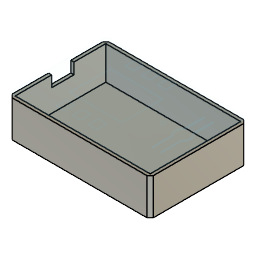
hamba gaming consol back shell (Autodesk Fusion 360 design; units mm, degrees)
Autodesk Fusion 360 part; units mm, degrees
sketch "Sketch1" plane through (0, 0, 0) normal (0, 0, 1) x (1, 0, 0)
  line L0 (0, 0) -> (83, 0)
  line L1 (83, 0) -> (83, 55)
  line L2 (83, 55) -> (0, 55)
  line L3 (0, 55) -> (0, 0)
  dimension "d1" = 83
  dimension "d2" = 55
  constraint horizontal L0
  constraint vertical L1
  constraint horizontal L2
  constraint vertical L3
  constraint coincident L0.start L3.end
  measures "d1" distance of L0.start L0.end
  measures "d2" distance of L0.start L2.end
extrude "Extrude1" add sketch "Sketch1" along normal blind 10 makes body 1
sketch "Sketch2" plane through (0, 0, 10) normal (0, 0, 1) x (-1, 0, 0)
  line L0 (0, -55) -> (0, 0)
  line L1 (0, 0) -> (-83, 0)
  line L2 (-83, 0) -> (-83, -55)
  line L3 (-83, -55) -> (0, -55)
  line L4 (-49, -42) -> (-49, -37.6986)
  line L5 (-49, -37.6986) -> (-52.5265, -34.3884)
  line L6 (-52.5265, -34.3884) -> (-52.5265, -24)
  line L7 (-52.5265, -24) -> (-49, -20.2432)
  line L8 (-49, -20.2432) -> (-49, -16)
  line L9 (-49, -16) -> (-2, -16)
  line L10 (-2, -16) -> (-0.5319, -18.1216)
  line L11 (-0.5319, -18.1216) -> (-0.5319, -23)
  line L12 (-0.5319, -23) -> (-1.2659, -24.8699)
  line L13 (-1.2659, -24.8699) -> (-1.2659, -33)
  line L14 (-1.2659, -33) -> (-0.5319, -34.4212)
  line L15 (-0.5319, -34.4212) -> (-0.5319, -39.5049)
  line L16 (-0.5319, -39.5049) -> (-3.3048, -42.6926)
  line L17 (-3.3048, -42.6926) -> (-49, -42)
  constraint perpendicular L5 L7
  constraint parallel L6 L8
  constraint perpendicular L0 L9
  constraint perpendicular L9 L11
  constraint parallel L11 L13
  constraint parallel L13 L15
  constraint vertical L4
extrude "Extrude2" add sketch "Sketch2" along normal blind 6 contours L4 L5 L6 L7 L8 L9 L10 L11 L12 L13 L14 L15 L16 L17 bodies 1
sketch "Sketch3" plane through (0, 0, 16) normal (0, 0, 1) x (-1, 0, 0)
  line L0 (-3.3048, -42.6926) -> (-0.5319, -39.5049)
  line L1 (-0.5319, -39.5049) -> (-0.5319, -34.4212)
  line L2 (-0.5319, -34.4212) -> (-1.2659, -33)
  line L3 (-1.2659, -33) -> (-1.2659, -24.8699)
  line L4 (-1.2659, -24.8699) -> (-0.5319, -23)
  line L5 (-0.5319, -23) -> (-0.5319, -18.1216)
  line L6 (-0.5319, -18.1216) -> (-2, -16)
  line L7 (-2, -16) -> (-49, -16)
  line L8 (-49, -16) -> (-49, -20.2432)
  line L9 (-49, -20.2432) -> (-52.5265, -24)
  line L10 (-52.5265, -24) -> (-52.5265, -34.3884)
  line L11 (-52.5265, -34.3884) -> (-49, -37.6986)
  line L12 (-49, -37.6986) -> (-49, -42)
  line L13 (-49, -42) -> (-3.3048, -42.6926)
  line L14 (-46, -38) -> (-20, -38)
  line L15 (-20, -38) -> (-20, -20)
  line L16 (-20, -20) -> (-46, -20)
  line L17 (-46, -20) -> (-46, -38)
  constraint horizontal L14
  constraint vertical L15
  constraint horizontal L16
  constraint vertical L17
extrude "Extrude3" add sketch "Sketch3" along normal blind 5 contours L14 L15 L16 L17 bodies 1
sketch "Sketch4" plane through (0, 0, 16) normal (0, 0, 1) x (-1, 0, 0)
  line L0 (-46, -20) -> (-20, -20)
  line L1 (-20, -20) -> (-20, -38)
  line L2 (-20, -38) -> (-46, -38)
  line L3 (-46, -38) -> (-46, -20)
  line L4 (-3.3048, -42.6926) -> (-0.5319, -39.5049)
  line L5 (-0.5319, -39.5049) -> (-0.5319, -34.4212)
  line L6 (-0.5319, -34.4212) -> (-1.2659, -33)
  line L7 (-1.2659, -33) -> (-1.2659, -24.8699)
  line L8 (-1.2659, -24.8699) -> (-0.5319, -23)
  line L9 (-0.5319, -23) -> (-0.5319, -18.1216)
  line L10 (-0.5319, -18.1216) -> (-2, -16)
  line L11 (-2, -16) -> (-49, -16)
  line L12 (-49, -16) -> (-49, -20.2432)
  line L13 (-49, -20.2432) -> (-52.5265, -24)
  line L14 (-52.5265, -24) -> (-52.5265, -34.3884)
  line L15 (-52.5265, -34.3884) -> (-49, -37.6986)
  line L16 (-49, -37.6986) -> (-49, -42)
  line L17 (-49, -42) -> (-3.3048, -42.6926)
  line L18 (-1.2659, -33) -> (-7, -33)
  line L19 (-7, -33) -> (-7, -25)
  line L20 (-7, -25) -> (-1.2659, -25)
  line L21 (-1.2659, -25) -> (-1.2659, -33)
  constraint horizontal L18
  constraint vertical L19
  constraint horizontal L20
  constraint vertical L21
  constraint coincident L6.end L7.start
extrude "Extrude4" add sketch "Sketch4" along normal blind 2 contours L7 L18 L19 L20 L21 bodies 1
sketch "Sketch5" plane through (0, 0, 10) normal (0, 0, 1) x (-1, 0, 0)
  line L0 (-3.3048, -42.6926) -> (-49, -42)
  line L1 (-49, -42) -> (-49, -37.6986)
  line L2 (-49, -37.6986) -> (-52.5265, -34.3884)
  line L3 (-52.5265, -34.3884) -> (-52.5265, -24)
  line L4 (-52.5265, -24) -> (-49, -20.2432)
  line L5 (-49, -20.2432) -> (-49, -16)
  line L6 (-49, -16) -> (-2, -16)
  line L7 (-2, -16) -> (-0.5319, -18.1216)
  line L8 (-0.5319, -18.1216) -> (-0.5319, -23)
  line L9 (-0.5319, -23) -> (-1.2659, -24.8699)
  line L10 (-1.2659, -24.8699) -> (-1.2659, -33)
  line L11 (-1.2659, -33) -> (-0.5319, -34.4212)
  line L12 (-0.5319, -34.4212) -> (-0.5319, -39.5049)
  line L13 (-0.5319, -39.5049) -> (-3.3048, -42.6926)
  line L14 (0, -55) -> (0, 0)
  line L15 (0, 0) -> (-83, 0)
  line L16 (-83, 0) -> (-83, -55)
  line L17 (-83, -55) -> (0, -55)
  line L18 (-43.127, -5.4877) -> (-41.627, -5.4877)
  line L19 (-40.877, -6.2377) -> (-40.877, -8.8377)
  line L20 (-41.627, -9.5877) -> (-43.127, -9.5877)
  line L21 (-43.877, -8.8377) -> (-43.877, -6.2377)
  arc A0 (-43.127, -5.4877) -> (-43.877, -6.2377) centre (-43.127, -6.2377) ccw
  arc A1 (-40.877, -6.2377) -> (-41.627, -5.4877) centre (-41.627, -6.2377) ccw
  arc A2 (-41.627, -9.5877) -> (-40.877, -8.8377) centre (-41.627, -8.8377) ccw
  arc A3 (-43.877, -8.8377) -> (-43.127, -9.5877) centre (-43.127, -8.8377) ccw
  arc A4 (-31.377, -9.5877) -> (-30.627, -8.8377) centre (-31.377, -8.8377) ccw
  line L22 (-31.377, -9.5877) -> (-32.877, -9.5877)
  arc A5 (-33.627, -8.8377) -> (-32.877, -9.5877) centre (-32.877, -8.8377) ccw
  line L23 (-33.627, -8.8377) -> (-33.627, -6.2377)
  arc A6 (-32.877, -5.4877) -> (-33.627, -6.2377) centre (-32.877, -6.2377) ccw
  line L24 (-32.877, -5.4877) -> (-31.377, -5.4877)
  arc A7 (-30.627, -6.2377) -> (-31.377, -5.4877) centre (-31.377, -6.2377) ccw
  line L25 (-30.627, -6.2377) -> (-30.627, -8.8377)
  arc A8 (-21.127, -9.5877) -> (-20.377, -8.8377) centre (-21.127, -8.8377) ccw
  line L26 (-21.127, -9.5877) -> (-22.627, -9.5877)
  arc A9 (-23.377, -8.8377) -> (-22.627, -9.5877) centre (-22.627, -8.8377) ccw
  line L27 (-23.377, -8.8377) -> (-23.377, -6.2377)
  arc A10 (-22.627, -5.4877) -> (-23.377, -6.2377) centre (-22.627, -6.2377) ccw
  line L28 (-22.627, -5.4877) -> (-21.127, -5.4877)
  arc A11 (-20.377, -6.2377) -> (-21.127, -5.4877) centre (-21.127, -6.2377) ccw
  line L29 (-20.377, -6.2377) -> (-20.377, -8.8377)
  arc A12 (-41.627, -53.0877) -> (-40.877, -52.3377) centre (-41.627, -52.3377) ccw
  line L30 (-41.627, -53.0877) -> (-43.127, -53.0877)
  arc A13 (-43.877, -52.3377) -> (-43.127, -53.0877) centre (-43.127, -52.3377) ccw
  line L31 (-43.877, -52.3377) -> (-43.877, -49.7377)
  arc A14 (-43.127, -48.9877) -> (-43.877, -49.7377) centre (-43.127, -49.7377) ccw
  line L32 (-43.127, -48.9877) -> (-41.627, -48.9877)
  arc A15 (-40.877, -49.7377) -> (-41.627, -48.9877) centre (-41.627, -49.7377) ccw
  line L33 (-40.877, -49.7377) -> (-40.877, -52.3377)
  arc A16 (-31.377, -53.0877) -> (-30.627, -52.3377) centre (-31.377, -52.3377) ccw
  line L34 (-31.377, -53.0877) -> (-32.877, -53.0877)
  arc A17 (-33.627, -52.3377) -> (-32.877, -53.0877) centre (-32.877, -52.3377) ccw
  line L35 (-33.627, -52.3377) -> (-33.627, -49.7377)
  arc A18 (-32.877, -48.9877) -> (-33.627, -49.7377) centre (-32.877, -49.7377) ccw
  line L36 (-32.877, -48.9877) -> (-31.377, -48.9877)
  arc A19 (-30.627, -49.7377) -> (-31.377, -48.9877) centre (-31.377, -49.7377) ccw
  line L37 (-30.627, -49.7377) -> (-30.627, -52.3377)
  arc A20 (-21.127, -53.0877) -> (-20.377, -52.3377) centre (-21.127, -52.3377) ccw
  line L38 (-21.127, -53.0877) -> (-22.627, -53.0877)
  arc A21 (-23.377, -52.3377) -> (-22.627, -53.0877) centre (-22.627, -52.3377) ccw
  line L39 (-23.377, -52.3377) -> (-23.377, -49.7377)
  arc A22 (-22.627, -48.9877) -> (-23.377, -49.7377) centre (-22.627, -49.7377) ccw
  line L40 (-22.627, -48.9877) -> (-21.127, -48.9877)
  arc A23 (-20.377, -49.7377) -> (-21.127, -48.9877) centre (-21.127, -49.7377) ccw
  line L41 (-20.377, -49.7377) -> (-20.377, -52.3377)
  point P0 (-43.877, -5.4877)
  point P1 (-40.877, -5.4877)
  point P2 (-43.877, -9.5877)
  dimension "d11" = 3
  dimension "d12" = 4.1
  dimension "d13" = 0.75
  dimension "d16" = 20.5
  dimension "d17" = -43.5
  constraint horizontal L18
  constraint vertical L19
  constraint horizontal L20
  constraint vertical L21
  constraint coincident P0 L21
  constraint coincident P0 L18
  constraint tangent L21 A0
  constraint tangent L18 A0
  constraint coincident P1 L19
  constraint coincident P1 L18
  constraint tangent L19 A1
  constraint tangent L18 A1
  constraint equal A0 A1
  constraint tangent L20 A2
  constraint tangent L19 A2
  constraint equal A0 A2
  constraint coincident P2 L21
  constraint coincident P2 L20
  constraint tangent L21 A3
  constraint tangent L20 A3
  constraint equal A0 A3
  measures "d11" distance of P0 P1
  measures "d12" distance of P0 P2
  measures "d13" radius of A0
extrude "Extrude5" add sketch "Sketch5" along normal blind 10 contours L18 L19 L20 L21 A0 A1 A2 A3 | A4 L22 A5 L23 A6 L24 A7 L25 | A8 L26 A9 L27 A10 L28 A11 L29 | A12 L30 A13 L31 A14 L32 A15 L33 | A16 L34 A17 L35 A18 L36 A19 L37 | A20 L38 A21 L39 A22 L40 A23 L41 bodies 1
sketch "Sketch6" plane through (0, 0, 10) normal (0, 0, 1) x (-1, 0, 0)
  line L0 (-43.127, -48.9877) -> (-41.627, -48.9877)
  arc A0 (-40.877, -49.7377) -> (-41.627, -48.9877) centre (-41.627, -49.7377) ccw
  line L1 (-40.877, -49.7377) -> (-40.877, -52.3377)
  arc A1 (-41.627, -53.0877) -> (-40.877, -52.3377) centre (-41.627, -52.3377) ccw
  line L2 (-41.627, -53.0877) -> (-43.127, -53.0877)
  arc A2 (-43.877, -52.3377) -> (-43.127, -53.0877) centre (-43.127, -52.3377) ccw
  line L3 (-43.877, -52.3377) -> (-43.877, -49.7377)
  arc A3 (-43.127, -48.9877) -> (-43.877, -49.7377) centre (-43.127, -49.7377) ccw
  line L4 (-32.877, -5.4877) -> (-31.377, -5.4877)
  arc A4 (-30.627, -6.2377) -> (-31.377, -5.4877) centre (-31.377, -6.2377) ccw
  line L5 (-30.627, -6.2377) -> (-30.627, -8.8377)
  arc A5 (-31.377, -9.5877) -> (-30.627, -8.8377) centre (-31.377, -8.8377) ccw
  line L6 (-31.377, -9.5877) -> (-32.877, -9.5877)
  arc A6 (-33.627, -8.8377) -> (-32.877, -9.5877) centre (-32.877, -8.8377) ccw
  line L7 (-33.627, -8.8377) -> (-33.627, -6.2377)
  arc A7 (-32.877, -5.4877) -> (-33.627, -6.2377) centre (-32.877, -6.2377) ccw
  line L8 (-22.627, -5.4877) -> (-21.127, -5.4877)
  arc A8 (-20.377, -6.2377) -> (-21.127, -5.4877) centre (-21.127, -6.2377) ccw
  line L9 (-20.377, -6.2377) -> (-20.377, -8.8377)
  arc A9 (-21.127, -9.5877) -> (-20.377, -8.8377) centre (-21.127, -8.8377) ccw
  line L10 (-21.127, -9.5877) -> (-22.627, -9.5877)
  arc A10 (-23.377, -8.8377) -> (-22.627, -9.5877) centre (-22.627, -8.8377) ccw
  line L11 (-23.377, -8.8377) -> (-23.377, -6.2377)
  arc A11 (-22.627, -5.4877) -> (-23.377, -6.2377) centre (-22.627, -6.2377) ccw
  line L12 (-32.877, -48.9877) -> (-31.377, -48.9877)
  arc A12 (-30.627, -49.7377) -> (-31.377, -48.9877) centre (-31.377, -49.7377) ccw
  line L13 (-30.627, -49.7377) -> (-30.627, -52.3377)
  arc A13 (-31.377, -53.0877) -> (-30.627, -52.3377) centre (-31.377, -52.3377) ccw
  line L14 (-31.377, -53.0877) -> (-32.877, -53.0877)
  arc A14 (-33.627, -52.3377) -> (-32.877, -53.0877) centre (-32.877, -52.3377) ccw
  line L15 (-33.627, -52.3377) -> (-33.627, -49.7377)
  arc A15 (-32.877, -48.9877) -> (-33.627, -49.7377) centre (-32.877, -49.7377) ccw
  line L16 (-43.127, -5.4877) -> (-41.627, -5.4877)
  arc A16 (-40.877, -6.2377) -> (-41.627, -5.4877) centre (-41.627, -6.2377) ccw
  line L17 (-40.877, -6.2377) -> (-40.877, -8.8377)
  arc A17 (-41.627, -9.5877) -> (-40.877, -8.8377) centre (-41.627, -8.8377) ccw
  line L18 (-41.627, -9.5877) -> (-43.127, -9.5877)
  arc A18 (-43.877, -8.8377) -> (-43.127, -9.5877) centre (-43.127, -8.8377) ccw
  line L19 (-43.877, -8.8377) -> (-43.877, -6.2377)
  arc A19 (-43.127, -5.4877) -> (-43.877, -6.2377) centre (-43.127, -6.2377) ccw
  line L20 (-22.627, -48.9877) -> (-21.127, -48.9877)
  arc A20 (-20.377, -49.7377) -> (-21.127, -48.9877) centre (-21.127, -49.7377) ccw
  line L21 (-20.377, -49.7377) -> (-20.377, -52.3377)
  arc A21 (-21.127, -53.0877) -> (-20.377, -52.3377) centre (-21.127, -52.3377) ccw
  line L22 (-21.127, -53.0877) -> (-22.627, -53.0877)
  arc A22 (-23.377, -52.3377) -> (-22.627, -53.0877) centre (-22.627, -52.3377) ccw
  line L23 (-23.377, -52.3377) -> (-23.377, -49.7377)
  arc A23 (-22.627, -48.9877) -> (-23.377, -49.7377) centre (-22.627, -49.7377) ccw
  line L24 (-3.3048, -42.6926) -> (-49, -42)
  line L25 (-49, -42) -> (-49, -37.6986)
  line L26 (-49, -37.6986) -> (-52.5265, -34.3884)
  line L27 (-52.5265, -34.3884) -> (-52.5265, -24)
  line L28 (-52.5265, -24) -> (-49, -20.2432)
  line L29 (-49, -20.2432) -> (-49, -16)
  line L30 (-49, -16) -> (-2, -16)
  line L31 (-2, -16) -> (-0.5319, -18.1216)
  line L32 (-0.5319, -18.1216) -> (-0.5319, -23)
  line L33 (-0.5319, -23) -> (-1.2659, -24.8699)
  line L34 (-1.2659, -24.8699) -> (-1.2659, -33)
  line L35 (-1.2659, -33) -> (-0.5319, -34.4212)
  line L36 (-0.5319, -34.4212) -> (-0.5319, -39.5049)
  line L37 (-0.5319, -39.5049) -> (-3.3048, -42.6926)
  line L38 (0, -55) -> (0, 0)
  line L39 (0, 0) -> (-83, 0)
  line L40 (-83, 0) -> (-83, -55)
  line L41 (-83, -55) -> (0, -55)
  circle A24 centre (-62, -29) radius 6
  dimension "d20" = 12
  measures "d20" diameter of A24
extrude "Extrude6" add sketch "Sketch6" along normal blind 10 contours A24 bodies 1
sketch "Sketch7" plane through (0, 0, 10) normal (0, 0, 1) x (-1, 0, 0)
  circle A0 centre (-62, -29) radius 6
  line L0 (-43.127, -48.9877) -> (-41.627, -48.9877)
  arc A1 (-40.877, -49.7377) -> (-41.627, -48.9877) centre (-41.627, -49.7377) ccw
  line L1 (-40.877, -49.7377) -> (-40.877, -52.3377)
  arc A2 (-41.627, -53.0877) -> (-40.877, -52.3377) centre (-41.627, -52.3377) ccw
  line L2 (-41.627, -53.0877) -> (-43.127, -53.0877)
  arc A3 (-43.877, -52.3377) -> (-43.127, -53.0877) centre (-43.127, -52.3377) ccw
  line L3 (-43.877, -52.3377) -> (-43.877, -49.7377)
  arc A4 (-43.127, -48.9877) -> (-43.877, -49.7377) centre (-43.127, -49.7377) ccw
  line L4 (-32.877, -5.4877) -> (-31.377, -5.4877)
  arc A5 (-30.627, -6.2377) -> (-31.377, -5.4877) centre (-31.377, -6.2377) ccw
  line L5 (-30.627, -6.2377) -> (-30.627, -8.8377)
  arc A6 (-31.377, -9.5877) -> (-30.627, -8.8377) centre (-31.377, -8.8377) ccw
  line L6 (-31.377, -9.5877) -> (-32.877, -9.5877)
  arc A7 (-33.627, -8.8377) -> (-32.877, -9.5877) centre (-32.877, -8.8377) ccw
  line L7 (-33.627, -8.8377) -> (-33.627, -6.2377)
  arc A8 (-32.877, -5.4877) -> (-33.627, -6.2377) centre (-32.877, -6.2377) ccw
  line L8 (-22.627, -5.4877) -> (-21.127, -5.4877)
  arc A9 (-20.377, -6.2377) -> (-21.127, -5.4877) centre (-21.127, -6.2377) ccw
  line L9 (-20.377, -6.2377) -> (-20.377, -8.8377)
  arc A10 (-21.127, -9.5877) -> (-20.377, -8.8377) centre (-21.127, -8.8377) ccw
  line L10 (-21.127, -9.5877) -> (-22.627, -9.5877)
  arc A11 (-23.377, -8.8377) -> (-22.627, -9.5877) centre (-22.627, -8.8377) ccw
  line L11 (-23.377, -8.8377) -> (-23.377, -6.2377)
  arc A12 (-22.627, -5.4877) -> (-23.377, -6.2377) centre (-22.627, -6.2377) ccw
  line L12 (-32.877, -48.9877) -> (-31.377, -48.9877)
  arc A13 (-30.627, -49.7377) -> (-31.377, -48.9877) centre (-31.377, -49.7377) ccw
  line L13 (-30.627, -49.7377) -> (-30.627, -52.3377)
  arc A14 (-31.377, -53.0877) -> (-30.627, -52.3377) centre (-31.377, -52.3377) ccw
  line L14 (-31.377, -53.0877) -> (-32.877, -53.0877)
  arc A15 (-33.627, -52.3377) -> (-32.877, -53.0877) centre (-32.877, -52.3377) ccw
  line L15 (-33.627, -52.3377) -> (-33.627, -49.7377)
  arc A16 (-32.877, -48.9877) -> (-33.627, -49.7377) centre (-32.877, -49.7377) ccw
  line L16 (-43.127, -5.4877) -> (-41.627, -5.4877)
  arc A17 (-40.877, -6.2377) -> (-41.627, -5.4877) centre (-41.627, -6.2377) ccw
  line L17 (-40.877, -6.2377) -> (-40.877, -8.8377)
  arc A18 (-41.627, -9.5877) -> (-40.877, -8.8377) centre (-41.627, -8.8377) ccw
  line L18 (-41.627, -9.5877) -> (-43.127, -9.5877)
  arc A19 (-43.877, -8.8377) -> (-43.127, -9.5877) centre (-43.127, -8.8377) ccw
  line L19 (-43.877, -8.8377) -> (-43.877, -6.2377)
  arc A20 (-43.127, -5.4877) -> (-43.877, -6.2377) centre (-43.127, -6.2377) ccw
  line L20 (-22.627, -48.9877) -> (-21.127, -48.9877)
  arc A21 (-20.377, -49.7377) -> (-21.127, -48.9877) centre (-21.127, -49.7377) ccw
  line L21 (-20.377, -49.7377) -> (-20.377, -52.3377)
  arc A22 (-21.127, -53.0877) -> (-20.377, -52.3377) centre (-21.127, -52.3377) ccw
  line L22 (-21.127, -53.0877) -> (-22.627, -53.0877)
  arc A23 (-23.377, -52.3377) -> (-22.627, -53.0877) centre (-22.627, -52.3377) ccw
  line L23 (-23.377, -52.3377) -> (-23.377, -49.7377)
  arc A24 (-22.627, -48.9877) -> (-23.377, -49.7377) centre (-22.627, -49.7377) ccw
  line L24 (-3.3048, -42.6926) -> (-49, -42)
  line L25 (-49, -42) -> (-49, -37.6986)
  line L26 (-49, -37.6986) -> (-52.5265, -34.3884)
  line L27 (-52.5265, -34.3884) -> (-52.5265, -24)
  line L28 (-52.5265, -24) -> (-49, -20.2432)
  line L29 (-49, -20.2432) -> (-49, -16)
  line L30 (-49, -16) -> (-2, -16)
  line L31 (-2, -16) -> (-0.5319, -18.1216)
  line L32 (-0.5319, -18.1216) -> (-0.5319, -23)
  line L33 (-0.5319, -23) -> (-1.2659, -24.8699)
  line L34 (-1.2659, -24.8699) -> (-1.2659, -33)
  line L35 (-1.2659, -33) -> (-0.5319, -34.4212)
  line L36 (-0.5319, -34.4212) -> (-0.5319, -39.5049)
  line L37 (-0.5319, -39.5049) -> (-3.3048, -42.6926)
  line L38 (0, -55) -> (0, 0)
  line L39 (0, 0) -> (-83, 0)
  line L40 (-83, 0) -> (-83, -55)
  line L41 (-83, -55) -> (0, -55)
  line L42 (-78.1154, -25.6476) -> (-72, -25.6476)
  line L43 (-72, -25.6476) -> (-72, -33)
  line L44 (-72, -33) -> (-78.1154, -33)
  line L45 (-78.1154, -33) -> (-78.1154, -25.6476)
  constraint horizontal L42
  constraint vertical L43
  constraint horizontal L44
  constraint vertical L45
extrude "Extrude7" add sketch "Sketch7" along normal blind 4 contours L42 L43 L44 L45 bodies 1
sketch "Sketch8" plane through (0, 0, 14) normal (0, 0, 1) x (-1, 0, 0)
  line L0 (-78.1154, -33) -> (-72, -33)
  line L1 (-72, -33) -> (-72, -25.6476)
  line L2 (-72, -25.6476) -> (-78.1154, -25.6476)
  line L3 (-78.1154, -25.6476) -> (-78.1154, -33)
  circle A0 centre (-75.1516, -29.2779) radius 1.6
  dimension "d25" = 3.2
  measures "d25" diameter of A0
extrude "Extrude8" add sketch "Sketch8" along normal blind 1 contours A0 bodies 1
extrude "Extrude9" add 1 faces at (61, 29.553, 20) along direction (0, 0, 1) blind 1 on bodies 1 bodies 1
sketch "Sketch9" plane through (0, 0, 0) normal (0, 0, 1) x (1, 0, 0)
  line L0 (83.9442, 56) -> (83.9442, -1)
  line L1 (83.9442, -1) -> (-1, -1)
  line L2 (-1, -1) -> (-1, 56)
  line L3 (-1, 56) -> (83.9442, 56)
  line L4 (83.9442, -1) -> (-1, -1)
  line L5 (-1, -1) -> (-1, 56)
  line L6 (-1, 56) -> (83.9442, 56)
  line L7 (83.9442, 56) -> (83.9442, -1)
  line L8 (85.9442, -3) -> (-3, -3)
  line L9 (-3, -3) -> (-3, 58)
  line L10 (-3, 58) -> (85.9442, 58)
  line L11 (85.9442, 58) -> (85.9442, -3)
  dimension "d31" = 0
  dimension "d32" = -2
  measures "d31" distance of L1
extrude "Extrude10" add sketch "Sketch9" along normal blind 19 separate body makes body 2
move_body "Move1" bodies 2 to x (1, 0, 0) y (0, 1, 0) z (0, 0, 1) at (0, 0, 2)
extrude "Extrude11" add 1 faces at (55.6295, -2.3333, 2) along direction (0, 0, -1) blind 4 on bodies 2 bodies 2
sketch "Sketch10" plane through (-1, 0, 0) normal (1, 0, 0) x (0, 1, 0)
  line L0 (56, -2) -> (56, 21)
  line L1 (56, 21) -> (-1, 21)
  line L2 (-1, 21) -> (-1, -2)
  line L3 (-1, -2) -> (56, -2)
  line L4 (-1, 0) -> (56, 0)
  dimension "d37" = -2
extrude "Extrude12" add sketch "Sketch10" along normal blind 84.944 contours L0 L2 L3 L4 bodies 2
extrude "Extrude13" cut 1 faces at (55.6295, -2.3333, 21) along direction (0, 0, -1) blind 2 on bodies 2 bodies 2
ref_plane "WorkPlane1" through (41.4721, 27.5, 19) normal (0, 0, -1) x (-1, 0, 0)
sketch "Sketch11" plane through (0, 0, 19) normal (0, 0, -1) x (-1, 0, 0)
  line L0 (3, 58) -> (-86, 58)
  line L1 (-86, 58) -> (-86, -3)
  line L2 (-86, -3) -> (3, -3)
  line L3 (3, -3) -> (3, 58)
  line L4 (-19.5019, 38.5864) -> (-45.906, 38.5864)
  line L5 (-45.906, 38.5864) -> (-45.906, 19.1931)
  line L6 (-45.906, 19.1931) -> (-19.5019, 19.1931)
  line L7 (-19.5019, 19.1931) -> (-19.5019, 38.5864)
  circle A0 centre (-62.1126, 28.8898) radius 1.4518
  line L8 (-20.2843, 53.1997) -> (-23.4767, 53.1997)
  line L9 (-23.4767, 53.1997) -> (-23.4767, 48.8872)
  line L10 (-23.4767, 48.8872) -> (-20.2843, 48.8872)
  line L11 (-20.2843, 48.8872) -> (-20.2843, 53.1997)
  line L12 (-30.5343, 48.8872) -> (-30.5343, 53.1997)
  line L13 (-30.5343, 53.1997) -> (-33.7267, 53.1997)
  line L14 (-33.7267, 53.1997) -> (-33.7267, 48.8872)
  line L15 (-33.7267, 48.8872) -> (-30.5343, 48.8872)
  line L16 (-40.7843, 48.8872) -> (-40.7843, 53.1997)
  line L17 (-40.7843, 53.1997) -> (-43.9767, 53.1997)
  line L18 (-43.9767, 53.1997) -> (-43.9767, 48.8872)
  line L19 (-43.9767, 48.8872) -> (-40.7843, 48.8872)
  line L20 (-20.2843, 5.3872) -> (-20.2843, 9.6997)
  line L21 (-20.2843, 9.6997) -> (-23.4767, 9.6997)
  line L22 (-23.4767, 9.6997) -> (-23.4767, 5.3872)
  line L23 (-23.4767, 5.3872) -> (-20.2843, 5.3872)
  line L24 (-30.5343, 5.3872) -> (-30.5343, 9.6997)
  line L25 (-30.5343, 9.6997) -> (-33.7267, 9.6997)
  line L26 (-33.7267, 9.6997) -> (-33.7267, 5.3872)
  line L27 (-33.7267, 5.3872) -> (-30.5343, 5.3872)
  line L28 (-40.7843, 5.3872) -> (-40.7843, 9.6997)
  line L29 (-40.7843, 9.6997) -> (-43.9767, 9.6997)
  line L30 (-43.9767, 9.6997) -> (-43.9767, 5.3872)
  line L31 (-43.9767, 5.3872) -> (-40.7843, 5.3872)
  dimension "d45" = -20.5
  dimension "d46" = -43.5
  constraint horizontal L0
  constraint vertical L1
  constraint horizontal L2
  constraint vertical L3
  constraint horizontal L4
  constraint vertical L5
  constraint horizontal L6
  constraint vertical L7
  constraint horizontal L8
  constraint vertical L9
  constraint horizontal L10
  constraint vertical L11
extrude "Extrude14" add sketch "Sketch11" against normal blind 2 separate body makes body 3
fillet "Fillet1" radius 1 24 edges at (23.4767, 51.0434, 21) (20.2843, 51.0434, 21) (21.8805, 53.1997, 21) (21.8805, 48.8872, 21) (30.5343, 51.0434, 21) (32.1305, 53.1997, 21) (33.7267, 51.0434, 21) (32.1305, 48.8872, 21) (40.7843, 51.0434, 21) (42.3805, 53.1997, 21) (43.9767, 51.0434, 21) (42.3805, 48.8872, 21) (21.8805, 9.6997, 21) (23.4767, 7.5434, 21) (20.2843, 7.5434, 21) (21.8805, 5.3872, 21) (32.1305, 5.3872, 21) (42.3805, 5.3872, 21) (40.7843, 7.5434, 21) (43.9767, 7.5434, 21) (42.3805, 9.6997, 21) (32.1305, 9.6997, 21) (30.5343, 7.5434, 21) (33.7267, 7.5434, 21) on bodies 3
fillet "Fillet2" radius 3.5 4 edges at (32.7039, 38.5864, 21) (19.5019, 28.8898, 21) (45.906, 28.8898, 21) (32.7039, 19.1931, 21) on bodies 3
sketch "Sketch12" plane through (0, 0, 21) normal (0, 0, 1) x (-1, 0, 0)
  line L0 (-39.7843, -10.6997) -> (-44.9767, -10.6997)
  line L1 (-44.9767, -10.6997) -> (-44.9767, -4.3872)
  line L2 (-44.9767, -4.3872) -> (-39.7843, -4.3872)
  line L3 (-39.7843, -4.3872) -> (-39.7843, -10.6997)
  line L4 (-24.4767, -4.3872) -> (-19.2843, -4.3872)
  line L5 (-19.2843, -4.3872) -> (-19.2843, -10.6997)
  line L6 (-19.2843, -10.6997) -> (-24.4767, -10.6997)
  line L7 (-24.4767, -10.6997) -> (-24.4767, -4.3872)
  line L8 (-34.7267, -54.1997) -> (-34.7267, -47.8872)
  line L9 (-34.7267, -47.8872) -> (-29.5343, -47.8872)
  line L10 (-29.5343, -47.8872) -> (-29.5343, -54.1997)
  line L11 (-29.5343, -54.1997) -> (-34.7267, -54.1997)
  line L12 (3, -58) -> (3, 3)
  line L13 (3, 3) -> (-86, 3)
  line L14 (-86, 3) -> (-86, -58)
  line L15 (-86, -58) -> (3, -58)
  circle A0 centre (-62.1126, -28.8898) radius 1.4518
  line L16 (-19.2843, -47.8872) -> (-19.2843, -54.1997)
  line L17 (-19.2843, -54.1997) -> (-24.4767, -54.1997)
  line L18 (-24.4767, -54.1997) -> (-24.4767, -47.8872)
  line L19 (-24.4767, -47.8872) -> (-19.2843, -47.8872)
  line L20 (-44.9767, -54.1997) -> (-44.9767, -47.8872)
  line L21 (-44.9767, -47.8872) -> (-39.7843, -47.8872)
  line L22 (-39.7843, -47.8872) -> (-39.7843, -54.1997)
  line L23 (-39.7843, -54.1997) -> (-44.9767, -54.1997)
  line L24 (-29.5343, -10.6997) -> (-34.7267, -10.6997)
  line L25 (-34.7267, -10.6997) -> (-34.7267, -4.3872)
  line L26 (-34.7267, -4.3872) -> (-29.5343, -4.3872)
  line L27 (-29.5343, -4.3872) -> (-29.5343, -10.6997)
  line L28 (-49.0682, -16.0309) -> (-16.3397, -16.0309)
  line L29 (-16.3397, -16.0309) -> (-16.3397, -41.7487)
  line L30 (-16.3397, -41.7487) -> (-49.0682, -41.7487)
  line L31 (-49.0682, -41.7487) -> (-49.0682, -16.0309)
  line L32 (-72, -45) -> (-78, -45)
  line L33 (-78, -45) -> (-78, -12)
  line L34 (-78, -12) -> (-72, -12)
  line L35 (-72, -12) -> (-72, -45)
  circle A1 centre (-75, -28.5) radius 5
  dimension "d53" = 10
  constraint horizontal L32
  constraint vertical L33
  constraint horizontal L34
  constraint vertical L35
  measures "d53" diameter of A1
extrude "Extrude15" cut sketch "Sketch12" against normal blind 2 contours L32 L33 L35 A1 | L33 L35 A1 | L35 A1 | L33 A1 | L33 L34 L35 A1 bodies 3
sketch "Sketch13" plane through (0, 45, 0) normal (0, -1, 0) x (1, 0, 0)
  line L0 (78, 21) -> (72, 21)
  line L1 (72, 21) -> (72, 19)
  line L2 (72, 19) -> (78, 19)
  line L3 (78, 19) -> (78, 21)
  line L4 (72.5, 21) -> (72.5, 19)
  line L5 (77.5, 19) -> (77.5, 21)
  dimension "d56" = -0.5
  dimension "d57" = -0.5
extrude "Extrude16" add sketch "Sketch13" along normal blind 33 contours L0 L2 L4 L5 bodies 3
sketch "Sketch14" plane through (0, 0, 21) normal (0, 0, 1) x (-1, 0, 0)
  line L0 (-72.5, -12) -> (-72, -12)
  line L1 (-72, -12) -> (-72, -24.5)
  arc A0 (-72, -32.5) -> (-72, -24.5) centre (-75, -28.5) ccw
  line L2 (-72, -32.5) -> (-72, -45)
  line L3 (-72, -45) -> (-72.5, -45)
  line L4 (-72.5, -45) -> (-72.5, -12)
  line L5 (-77.5, -12) -> (-77.5, -45)
  line L6 (-77.5, -45) -> (-78, -45)
  line L7 (-78, -45) -> (-78, -32.5)
  arc A1 (-78, -24.5) -> (-78, -32.5) centre (-75, -28.5) ccw
  line L8 (-78, -24.5) -> (-78, -12)
  line L9 (-78, -12) -> (-77.5, -12)
  line L10 (-39.7843, -10.6997) -> (-44.9767, -10.6997)
  line L11 (-44.9767, -10.6997) -> (-44.9767, -4.3872)
  line L12 (-44.9767, -4.3872) -> (-39.7843, -4.3872)
  line L13 (-39.7843, -4.3872) -> (-39.7843, -10.6997)
  line L14 (-24.4767, -4.3872) -> (-19.2843, -4.3872)
  line L15 (-19.2843, -4.3872) -> (-19.2843, -10.6997)
  line L16 (-19.2843, -10.6997) -> (-24.4767, -10.6997)
  line L17 (-24.4767, -10.6997) -> (-24.4767, -4.3872)
  line L18 (-34.7267, -54.1997) -> (-34.7267, -47.8872)
  line L19 (-34.7267, -47.8872) -> (-29.5343, -47.8872)
  line L20 (-29.5343, -47.8872) -> (-29.5343, -54.1997)
  line L21 (-29.5343, -54.1997) -> (-34.7267, -54.1997)
  line L22 (3, -58) -> (3, 3)
  line L23 (3, 3) -> (-86, 3)
  line L24 (-86, 3) -> (-86, -58)
  line L25 (-86, -58) -> (3, -58)
  circle A2 centre (-62.1126, -28.8898) radius 1.4518
  line L26 (-19.2843, -47.8872) -> (-19.2843, -54.1997)
  line L27 (-19.2843, -54.1997) -> (-24.4767, -54.1997)
  line L28 (-24.4767, -54.1997) -> (-24.4767, -47.8872)
  line L29 (-24.4767, -47.8872) -> (-19.2843, -47.8872)
  line L30 (-44.9767, -54.1997) -> (-44.9767, -47.8872)
  line L31 (-44.9767, -47.8872) -> (-39.7843, -47.8872)
  line L32 (-39.7843, -47.8872) -> (-39.7843, -54.1997)
  line L33 (-39.7843, -54.1997) -> (-44.9767, -54.1997)
  line L34 (-29.5343, -10.6997) -> (-34.7267, -10.6997)
  line L35 (-34.7267, -10.6997) -> (-34.7267, -4.3872)
  line L36 (-34.7267, -4.3872) -> (-29.5343, -4.3872)
  line L37 (-29.5343, -4.3872) -> (-29.5343, -10.6997)
  line L38 (-49.0682, -16.0309) -> (-16.3397, -16.0309)
  line L39 (-16.3397, -16.0309) -> (-16.3397, -41.7487)
  line L40 (-16.3397, -41.7487) -> (-49.0682, -41.7487)
  line L41 (-49.0682, -41.7487) -> (-49.0682, -16.0309)
  circle A3 centre (-75, -28.5) radius 4.25
  dimension "d60" = 8.5
  constraint concentric A0 A3
  measures "d60" diameter of A3
extrude "Extrude17" add sketch "Sketch14" against normal blind 2 contours L4 A3 | L5 A3 bodies 3
move_body "Move2" bodies 3 to x (1, 0, 0) y (0, 1, 0) z (0, 0, 1) at (0, 0, 2)
extrude "Extrude18" add 1 faces at (74.819, 28.3981, 15) along direction (0, 0, 1) blind 8 separate body on bodies 1 makes body 4
combine "Combine1" operation add target body 3 tool bodies 4
extrude "Extrude19" cut 1 faces at (74.819, 28.3981, 15) along direction (0, 0, 1) blind 0.3 on bodies 3 bodies 3
move_face "MoveFace1" to x (1, 0, 0) y (0, 1, 0) z (0, 0, 1) at (0, -0.6, 0) 2 faces at (74.819, 28.3981, 15.3) (75.1117, 27.6783, 19.1) on bodies 3
fillet "Fillet3" radius 2 1 edges at (76.6433, 29.2564, 21) on bodies 3
extrude "Extrude20" add 1 faces at (55.6295, -2.3333, 19) along direction (0, 0, 1) blind 2 on bodies 2 bodies 2
chamfer "Chamfer1" distance 2 angle 45 4 edges at (-3, 58, 9.5) (-3, -3, 9.5) (85.9442, -3, 9.5) (85.9442, 58, 9.5) on bodies 2
chamfer "Chamfer2" distance 2 angle 45 4 edges at (86, -3, 22) (86, 58, 22) (-3, -3, 22) (-3, 58, 22) on bodies 3
sketch "Sketch15" plane through (1.2659, 0, 0) normal (-1, 0, 0) x (0, -1, 0)
  line L0 (-33, 10) -> (-24.8699, 10)
  line L1 (-24.8699, 10) -> (-24.8699, 16)
  line L2 (-24.8699, 16) -> (-25, 16)
  line L3 (-25, 16) -> (-25, 18)
  line L4 (-25, 18) -> (-33, 18)
  line L5 (-33, 18) -> (-33, 16)
  line L6 (-33, 16) -> (-33, 10)
  line L7 (-33, 16) -> (-25, 16)
  constraint coincident L5.end L6.start
  constraint coincident L2.end L3.start
extrude "Extrude21" add sketch "Sketch15" along normal blind 4.266 separate body contours L3 L4 L5 L7 makes body 5
sketch "Sketch16" plane through (-3, 0, 0) normal (-1, 0, 0) x (0, -1, 0)
  line L0 (1, -2) -> (1, 21)
  line L1 (1, 21) -> (-56, 21)
  line L2 (-56, 21) -> (-56, -2)
  line L3 (-56, -2) -> (1, -2)
  line L4 (-22, 21) -> (-22, 14)
  line L5 (-22, 14) -> (-36, 14)
  line L6 (-36, 14) -> (-36, 21)
  constraint vertical L4
  constraint horizontal L5
  constraint vertical L6
  constraint coincident L1 L6.end
  constraint coincident L1 L4.start
delete_body "RemoveBody1" bodies 5
extrude "Extrude22" cut sketch "Sketch16" against normal blind 2 contours L1 L4 L5 L6 bodies 2
sketch "Sketch17" plane through (0, 0, 21) normal (0, 0, -1) x (1, 0, 0)
  circle A0 centre (75.1516, -28.6779) radius 3.6
  line L0 (77.5, -12) -> (78, -12)
  line L1 (78, -12) -> (78, -24.5)
  arc A1 (78, -32.5) -> (78, -24.5) centre (75, -28.5) ccw
  line L2 (78, -32.5) -> (78, -45)
  line L3 (78, -45) -> (77.5, -45)
  line L4 (77.5, -45) -> (77.5, -31.9369)
  arc A2 (77.5, -31.9369) -> (77.5, -25.0631) centre (75, -28.5) ccw
  line L5 (77.5, -25.0631) -> (77.5, -12)
  line L6 (72.5, -31.9369) -> (72.5, -45)
  line L7 (72.5, -45) -> (72, -45)
  line L8 (72, -45) -> (72, -32.5)
  arc A3 (72, -24.5) -> (72, -32.5) centre (75, -28.5) ccw
  line L9 (72, -24.5) -> (72, -12)
  line L10 (72, -12) -> (72.5, -12)
  line L11 (72.5, -12) -> (72.5, -25.0631)
  arc A4 (72.5, -25.0631) -> (72.5, -31.9369) centre (75, -28.5) ccw
  line L12 (40.7843, -5.3872) -> (43.9767, -5.3872)
  line L13 (43.9767, -5.3872) -> (43.9767, -9.6997)
  line L14 (43.9767, -9.6997) -> (40.7843, -9.6997)
  line L15 (40.7843, -9.6997) -> (40.7843, -5.3872)
  line L16 (30.5343, -48.8872) -> (33.7267, -48.8872)
  line L17 (33.7267, -48.8872) -> (33.7267, -53.1997)
  line L18 (33.7267, -53.1997) -> (30.5343, -53.1997)
  line L19 (30.5343, -53.1997) -> (30.5343, -48.8872)
  line L20 (40.7843, -48.8872) -> (43.9767, -48.8872)
  line L21 (43.9767, -48.8872) -> (43.9767, -53.1997)
  line L22 (43.9767, -53.1997) -> (40.7843, -53.1997)
  line L23 (40.7843, -53.1997) -> (40.7843, -48.8872)
  line L24 (20.2843, -5.3872) -> (23.4767, -5.3872)
  line L25 (23.4767, -5.3872) -> (23.4767, -9.6997)
  line L26 (23.4767, -9.6997) -> (20.2843, -9.6997)
  line L27 (20.2843, -9.6997) -> (20.2843, -5.3872)
  line L28 (20.2843, -53.1997) -> (20.2843, -48.8872)
  line L29 (20.2843, -48.8872) -> (23.4767, -48.8872)
  line L30 (23.4767, -48.8872) -> (23.4767, -53.1997)
  line L31 (23.4767, -53.1997) -> (20.2843, -53.1997)
  line L32 (30.5343, -5.3872) -> (33.7267, -5.3872)
  line L33 (33.7267, -5.3872) -> (33.7267, -9.6997)
  line L34 (33.7267, -9.6997) -> (30.5343, -9.6997)
  line L35 (30.5343, -9.6997) -> (30.5343, -5.3872)
  circle A5 centre (62.1126, -28.8898) radius 1.4518
  line L36 (19.5019, -38.5864) -> (19.5019, -19.1931)
  line L37 (19.5019, -19.1931) -> (45.906, -19.1931)
  line L38 (45.906, -19.1931) -> (45.906, -38.5864)
  line L39 (45.906, -38.5864) -> (19.5019, -38.5864)
  line L40 (-3, -56) -> (-1, -58)
  line L41 (-1, -58) -> (84, -58)
  line L42 (84, -58) -> (86, -56)
  line L43 (86, -56) -> (86, 1)
  line L44 (86, 1) -> (84, 3)
  line L45 (84, 3) -> (-1, 3)
  line L46 (-1, 3) -> (-3, 1)
  line L47 (-3, 1) -> (-3, -56)
  line L48 (19.9843, -9.9997) -> (19.9843, -5.0872)
  line L49 (19.9843, -5.0872) -> (23.7767, -5.0872)
  line L50 (23.7767, -5.0872) -> (23.7767, -9.9997)
  line L51 (23.7767, -9.9997) -> (19.9843, -9.9997)
  line L52 (34.0267, -9.9997) -> (30.2343, -9.9997)
  line L53 (30.2343, -9.9997) -> (30.2343, -5.0872)
  line L54 (30.2343, -5.0872) -> (34.0267, -5.0872)
  line L55 (34.0267, -5.0872) -> (34.0267, -9.9997)
  line L56 (44.2767, -9.9997) -> (40.4843, -9.9997)
  line L57 (40.4843, -9.9997) -> (40.4843, -5.0872)
  line L58 (40.4843, -5.0872) -> (44.2767, -5.0872)
  line L59 (44.2767, -5.0872) -> (44.2767, -9.9997)
  line L60 (23.7767, -53.4997) -> (19.9843, -53.4997)
  line L61 (19.9843, -53.4997) -> (19.9843, -48.5872)
  line L62 (19.9843, -48.5872) -> (23.7767, -48.5872)
  line L63 (23.7767, -48.5872) -> (23.7767, -53.4997)
  line L64 (34.0267, -53.4997) -> (30.2343, -53.4997)
  line L65 (30.2343, -53.4997) -> (30.2343, -48.5872)
  line L66 (30.2343, -48.5872) -> (34.0267, -48.5872)
  line L67 (34.0267, -48.5872) -> (34.0267, -53.4997)
  line L68 (44.2767, -53.4997) -> (40.4843, -53.4997)
  line L69 (40.4843, -53.4997) -> (40.4843, -48.5872)
  line L70 (40.4843, -48.5872) -> (44.2767, -48.5872)
  line L71 (44.2767, -48.5872) -> (44.2767, -53.4997)
  dimension "d77" = -0.3
  dimension "d80" = 20.5
  dimension "d81" = -43.5
extrude "Extrude23" add sketch "Sketch17" along normal blind 0.5 contours L48 L49 L50 L51 | L52 L53 L54 L55 | L56 L57 L58 L59 | L60 L61 L62 L63 | L64 L65 L66 L67 | L68 L69 L70 L71 bodies 3
extrude "Extrude24" add 1 faces at (74.819, 27.7981, 15.3) along direction (0, 0, -1) blind 0.2 on bodies 3 bodies 3
sketch "Sketch18" plane through (0, 0, 21) normal (0, 0, -1) x (1, 0, 0)
  line L0 (44.2767, -48.5872) -> (44.2767, -53.4997)
  line L1 (44.2767, -53.4997) -> (40.4843, -53.4997)
  line L2 (40.4843, -53.4997) -> (40.4843, -48.5872)
  line L3 (40.4843, -48.5872) -> (44.2767, -48.5872)
  line L4 (34.0267, -5.0872) -> (34.0267, -9.9997)
  line L5 (34.0267, -9.9997) -> (30.2343, -9.9997)
  line L6 (30.2343, -9.9997) -> (30.2343, -5.0872)
  line L7 (30.2343, -5.0872) -> (34.0267, -5.0872)
  line L8 (44.2767, -5.0872) -> (44.2767, -9.9997)
  line L9 (44.2767, -9.9997) -> (40.4843, -9.9997)
  line L10 (40.4843, -9.9997) -> (40.4843, -5.0872)
  line L11 (40.4843, -5.0872) -> (44.2767, -5.0872)
  line L12 (34.0267, -48.5872) -> (34.0267, -53.4997)
  line L13 (34.0267, -53.4997) -> (30.2343, -53.4997)
  line L14 (30.2343, -53.4997) -> (30.2343, -48.5872)
  line L15 (30.2343, -48.5872) -> (34.0267, -48.5872)
  line L16 (23.7767, -9.9997) -> (19.9843, -9.9997)
  line L17 (19.9843, -9.9997) -> (19.9843, -5.0872)
  line L18 (19.9843, -5.0872) -> (23.7767, -5.0872)
  line L19 (23.7767, -5.0872) -> (23.7767, -9.9997)
  line L20 (23.7767, -48.5872) -> (23.7767, -53.4997)
  line L21 (23.7767, -53.4997) -> (19.9843, -53.4997)
  line L22 (19.9843, -53.4997) -> (19.9843, -48.5872)
  line L23 (19.9843, -48.5872) -> (23.7767, -48.5872)
  circle A0 centre (75.1516, -28.6779) radius 3.6
  line L24 (77.5, -12) -> (78, -12)
  line L25 (78, -12) -> (78, -24.5)
  arc A1 (78, -32.5) -> (78, -24.5) centre (75, -28.5) ccw
  line L26 (78, -32.5) -> (78, -45)
  line L27 (78, -45) -> (77.5, -45)
  line L28 (77.5, -45) -> (77.5, -31.9369)
  arc A2 (77.5, -31.9369) -> (77.5, -25.0631) centre (75, -28.5) ccw
  line L29 (77.5, -25.0631) -> (77.5, -12)
  line L30 (72.5, -31.9369) -> (72.5, -45)
  line L31 (72.5, -45) -> (72, -45)
  line L32 (72, -45) -> (72, -32.5)
  arc A3 (72, -24.5) -> (72, -32.5) centre (75, -28.5) ccw
  line L33 (72, -24.5) -> (72, -12)
  line L34 (72, -12) -> (72.5, -12)
  line L35 (72.5, -12) -> (72.5, -25.0631)
  arc A4 (72.5, -25.0631) -> (72.5, -31.9369) centre (75, -28.5) ccw
  circle A5 centre (62.1126, -28.8898) radius 1.4518
  line L36 (19.5019, -38.5864) -> (19.5019, -19.1931)
  line L37 (19.5019, -19.1931) -> (45.906, -19.1931)
  line L38 (45.906, -19.1931) -> (45.906, -38.5864)
  line L39 (45.906, -38.5864) -> (19.5019, -38.5864)
  line L40 (-3, -56) -> (-1, -58)
  line L41 (-1, -58) -> (84, -58)
  line L42 (84, -58) -> (86, -56)
  line L43 (86, -56) -> (86, 1)
  line L44 (86, 1) -> (84, 3)
  line L45 (84, 3) -> (-1, 3)
  line L46 (-1, 3) -> (-3, 1)
  line L47 (-3, 1) -> (-3, -56)
  line L48 (84, 1) -> (-1, 1)
  line L49 (-1, 1) -> (-1, 3)
  line L50 (84, 1) -> (84, 3)
  line L51 (-1, -56) -> (84, -56)
  line L52 (-1, -56) -> (-1, -58)
  line L53 (84, -56) -> (84, -58)
  dimension "d86" = -2
  dimension "d87" = -2
  constraint coincident L45.end L46.start
  constraint perpendicular L45 L49
  constraint coincident L44.end L45.start
  constraint perpendicular L45 L50
  constraint coincident L40.end L41.start
  constraint perpendicular L41 L52
  constraint coincident L41.end L42.start
  constraint perpendicular L41 L53
extrude "Extrude25" add sketch "Sketch18" along normal blind 8 contours L41 L51 L52 L53 | L45 L48 L49 L50 bodies 3
extrude "Extrude26" cut 2 faces at (84, -1.6667, 18.3333) (84, 56.6667, 18.3333) along direction (-1, 0, 0) blind 2 on bodies 3 bodies 3
extrude "Extrude27" cut 2 faces at (-1, 56.6667, 18.3333) (-1, -1.6667, 18.3333) along direction (1, 0, 0) blind 2 on bodies 3 bodies 3
sketch "Sketch19" plane through (0, -3, 0) normal (0, -1, 0) x (1, 0, 0)
  line L0 (-1, 21) -> (1, 21)
  line L1 (1, 21) -> (1, 13)
  line L2 (1, 13) -> (82, 13)
  line L3 (82, 13) -> (82, 21)
  line L4 (82, 21) -> (84, 21)
  line L5 (84, 21) -> (84, 23)
  line L6 (84, 23) -> (-1, 23)
  line L7 (-1, 23) -> (-1, 21)
  circle A0 centre (41.5, 13) radius 26.5
  ellipse E0 centre (41.5, 13) end of major axis (68, 13) minor radius 7
  line L8 (15, 13) -> (68, 13) construction
  line L9 (41.5, 6) -> (41.5, 20) construction
  dimension "d94" = 14
  constraint midpoint L2 A0.centre
  constraint coincident E0 L8.start
  constraint coincident E0 L8.end
  constraint coincident E0 L9.start
  constraint coincident E0 L9.end
  constraint concentric A0 E0
  constraint parallel L2 L8
extrude "Extrude28" cut sketch "Sketch19" against normal blind 79 contours L2 E0 picked at (41.6254, 15.3331) bodies 3
extrude "Extrude29" add 6 faces at (20.0843, 6.8247, 20.5) (30.3343, 6.8247, 20.5) (40.5843, 6.8247, 20.5) (40.5843, 50.3247, 20.5) (30.3343, 50.3247, 20.5) (20.0843, 50.3247, 20.5) along direction (0, 0, -1) blind 2 on bodies 3 bodies 3
extrude "Extrude30" add 1 faces at (5.7408, -1, 15.9683) along direction (0, 1, 0) blind 1.5 on bodies 3 bodies 3
sketch "Sketch20" plane through (0, -3, 0) normal (0, -1, 0) x (1, 0, 0)
  ellipse E0 centre (41.5, 13) end of major axis (68, 13) minor radius 7 (68, 13) -> (15, 13) ccw
  line L0 (68, 13) -> (82, 13)
  line L1 (82, 13) -> (82, 21)
  line L2 (82, 21) -> (84, 21)
  line L3 (84, 21) -> (84, 23)
  line L4 (84, 23) -> (-1, 23)
  line L5 (-1, 23) -> (-1, 21)
  line L6 (-1, 21) -> (1, 21)
  line L7 (1, 21) -> (1, 13)
  line L8 (1, 13) -> (15, 13)
  line L9 (1, 21) -> (82, 21)
  constraint coincident L6.end L7.start
  constraint coincident L1.end L2.start
extrude "Extrude31" cut sketch "Sketch20" against normal blind 2 contours E0 L0 L1 L7 L8 L9 bodies 3
extrude "Extrude32" add 1 faces at (5.7408, 56, 15.9683) along direction (0, -1, 0) blind 1.5 on bodies 3 bodies 3
sketch "Sketch21" plane through (0, 58, 0) normal (0, 1, 0) x (-1, 0, 0)
  ellipse E0 centre (-41.5, 13) end of major axis (-68, 13) minor radius 7 (-15, 13) -> (-68, 13) ccw
  line L0 (-15, 13) -> (-1, 13)
  line L1 (-1, 13) -> (-1, 21)
  line L2 (-1, 21) -> (1, 21)
  line L3 (1, 21) -> (1, 23)
  line L4 (1, 23) -> (-84, 23)
  line L5 (-84, 23) -> (-84, 21)
  line L6 (-84, 21) -> (-82, 21)
  line L7 (-82, 21) -> (-82, 13)
  line L8 (-82, 13) -> (-68, 13)
  line L9 (-82, 21) -> (-1, 21)
  constraint coincident L6.end L7.start
  constraint coincident L1.end L2.start
extrude "Extrude33" cut sketch "Sketch21" against normal blind 2 contours E0 L0 L1 L7 L8 L9 bodies 3
sketch "Sketch22" plane through (0, 0, 23) normal (0, 0, 1) x (-1, 0, 0)
  line L0 (1, -58) -> (3, -56)
  line L1 (3, -56) -> (3, 1)
  line L2 (3, 1) -> (1, 3)
  line L3 (1, 3) -> (-84, 3)
  line L4 (-84, 3) -> (-86, 1)
  line L5 (-86, 1) -> (-86, -56)
  line L6 (-86, -56) -> (-84, -58)
  line L7 (-84, -58) -> (1, -58)
  line L8 (-49.0682, -16.0309) -> (-16.3397, -16.0309)
  line L9 (-16.3397, -16.0309) -> (-16.3397, -41.7487)
  line L10 (-16.3397, -41.7487) -> (-49.0682, -41.7487)
  line L11 (-49.0682, -41.7487) -> (-49.0682, -16.0309)
  line L12 (-29.5343, -10.6997) -> (-34.7267, -10.6997)
  line L13 (-34.7267, -10.6997) -> (-34.7267, -4.3872)
  line L14 (-34.7267, -4.3872) -> (-29.5343, -4.3872)
  line L15 (-29.5343, -4.3872) -> (-29.5343, -10.6997)
  line L16 (-44.9767, -54.1997) -> (-44.9767, -47.8872)
  line L17 (-44.9767, -47.8872) -> (-39.7843, -47.8872)
  line L18 (-39.7843, -47.8872) -> (-39.7843, -54.1997)
  line L19 (-39.7843, -54.1997) -> (-44.9767, -54.1997)
  line L20 (-19.2843, -47.8872) -> (-19.2843, -54.1997)
  line L21 (-19.2843, -54.1997) -> (-24.4767, -54.1997)
  line L22 (-24.4767, -54.1997) -> (-24.4767, -47.8872)
  line L23 (-24.4767, -47.8872) -> (-19.2843, -47.8872)
  circle A0 centre (-62.1126, -28.8898) radius 1.4518
  line L24 (-34.7267, -54.1997) -> (-34.7267, -47.8872)
  line L25 (-34.7267, -47.8872) -> (-29.5343, -47.8872)
  line L26 (-29.5343, -47.8872) -> (-29.5343, -54.1997)
  line L27 (-29.5343, -54.1997) -> (-34.7267, -54.1997)
  line L28 (-24.4767, -4.3872) -> (-19.2843, -4.3872)
  line L29 (-19.2843, -4.3872) -> (-19.2843, -10.6997)
  line L30 (-19.2843, -10.6997) -> (-24.4767, -10.6997)
  line L31 (-24.4767, -10.6997) -> (-24.4767, -4.3872)
  line L32 (-39.7843, -10.6997) -> (-44.9767, -10.6997)
  line L33 (-44.9767, -10.6997) -> (-44.9767, -4.3872)
  line L34 (-44.9767, -4.3872) -> (-39.7843, -4.3872)
  line L35 (-39.7843, -4.3872) -> (-39.7843, -10.6997)
  line L36 (-77.5, -31.9369) -> (-77.5, -45)
  line L37 (-77.5, -45) -> (-78, -45)
  line L38 (-78, -45) -> (-78, -32.5)
  arc A1 (-78, -24.5) -> (-78, -32.5) centre (-75, -28.5) ccw
  line L39 (-78, -24.5) -> (-78, -12)
  line L40 (-78, -12) -> (-77.5, -12)
  line L41 (-77.5, -12) -> (-77.5, -25.0631)
  arc A2 (-77.5, -25.0631) -> (-77.5, -31.9369) centre (-75, -28.5) ccw
  line L42 (-72.5, -12) -> (-72, -12)
  line L43 (-72, -12) -> (-72, -24.5)
  arc A3 (-72, -32.5) -> (-72, -24.5) centre (-75, -28.5) ccw
  line L44 (-72, -32.5) -> (-72, -45)
  line L45 (-72, -45) -> (-72.5, -45)
  line L46 (-72.5, -45) -> (-72.5, -31.9369)
  arc A4 (-72.5, -31.9369) -> (-72.5, -25.0631) centre (-75, -28.5) ccw
  line L47 (-72.5, -25.0631) -> (-72.5, -12)
  dimension "d107" = 85
  dimension "d108" = 57
  dimension "d109" = 32.7286
  dimension "d110" = 25.7179
  dimension "d111" = 6.3125
  dimension "d112" = 2.9036
  dimension "d113" = 4.25
  dimension "d114" = 5
  dimension "d115" = 5
  dimension "d119" = 135
  measures "d107" distance of L0.start L6.end
  measures "d108" distance of L4.end L5.end
  measures "d109" distance of L9.end L10.end
  measures "d110" distance of L8.end L9.end
  measures "d111" distance of L20.start L20.end
  measures "d112" diameter of A0
  measures "d113" radius of A4
  measures "d114" radius of A3
  measures "d115" distance of L36.end L45.end
  measures "d119" angle of L0 L7
hidden bodies 1 3
named bodies: "Breadboard", "enclosure", "front cover"
